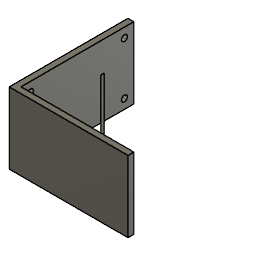
L_Bracket (Autodesk Fusion 360 design; units mm, degrees)
part number: 2026-08-27-11-16-52-339
Autodesk Fusion 360 part; units mm, degrees
note: some values were not read from the file. Chosen so that the rebuilt part matches the saved one: a direction.
sketch "Sketch1" plane through (0, 0, 0) normal (0, 1, 0) x (1, 0, 0)
  line L0 (0, 100) -> (0, 0)
  line L1 (0, 0) -> (100, 0)
  line L2 (100, 0) -> (100, 5)
  line L3 (100, 5) -> (5, 5)
  line L4 (5, 5) -> (5, 100)
  line L5 (5, 100) -> (0, 100)
  dimension "d1" = 100
  dimension "d2" = 100
  dimension "d3" = 95
  dimension "d4" = 5
  constraint coincident L0.end L1.start
  constraint vertical L0
  constraint perpendicular L0 L1
  constraint perpendicular L1 L2
  constraint perpendicular L2 L3
  constraint perpendicular L3 L4
  constraint perpendicular L0 L5
  measures "d1" distance of L0.end L1.end
  measures "d2" distance of L0.start L0.end
  measures "d3" distance of L2.end L3.end
  measures "d4" distance of L1.end L2.end
extrude "Extrude1" add sketch "Sketch1" along normal blind 60
sketch "Sketch2" plane through (5, 0, 0) normal (1, 0, 0) x (0, 0, -1)
  line L0 (5, 0) -> (100, 0)
  line L1 (100, 0) -> (100, 60)
  line L2 (100, 60) -> (5, 60)
  line L3 (5, 60) -> (5, 0)
  circle A0 centre (92, 8) radius 2.5
  circle A1 centre (92, 52) radius 2.5
  circle A2 centre (13, 8) radius 2.5
  circle A3 centre (13, 52) radius 2.5
  dimension "d15" = 5
  constraint equal A1 A3
  constraint equal A0 A1
  constraint equal A2 A3
  measures "d15" diameter of A3
extrude "Extrude2" cut sketch "Sketch2" against normal blind 5 contours A0 | A1 | A2 | A3
ref_plane "WorkPlane2" through (52.5, 30, -5) normal (0, -1, 0) x (1, 0, 0)
sketch "Sketch8" plane through (0, 30, 0) normal (0, -1, 0) x (-1, 0, 0)
  line L0 (-75, 5) -> (-5, 75)
rib "Rib1" add thickness 10 on both sides direction (-0.707107, 0, 0.707107) depth 2 extending the curves path "Sketch8" along L0
